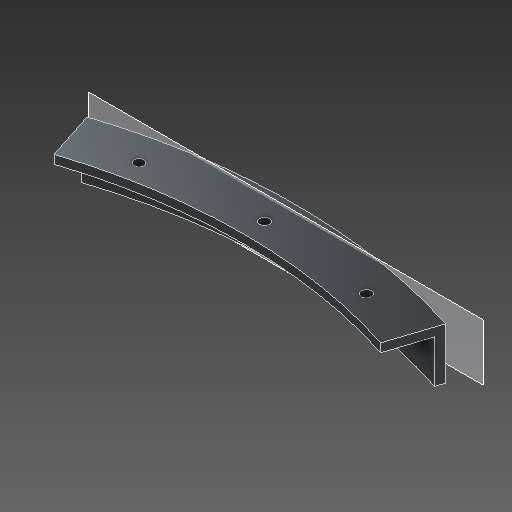
# Autodesk Inventor part: Casing_holder
Saved by Autodesk Inventor 2020 (Build 240168000, 168)
## iProperties
Created: 2022-08-25
Part Number: Casing_holder
Material: Iron, Gray Cast ASTM A48 Grade 60
Document SubType Name: Modeling
Designer: Umair
Density: 7.3953 g/cm^3
Appearance: Iron Gray
Author: Umair
Autodesk Inventor part; units mm, degrees
ref_plane "YZ Plane" through (0, 0, 0) normal (1, 0, 0) x (0, 1, 0)
ref_plane "XZ Plane" through (0, 0, 0) normal (0, 1, 0) x (-1, 0, 0)
sketch "Sketch1" plane through (0, 0, 0) normal (0, 1, 0) x (-1, 0, 0)
  circle A0 centre (0, 0) radius 200
  line L0 (0, 0) -> (0, -200)
  line L1 (0, 0) -> (-61.8034, -190.2113)
  line L2 (0, 0) -> (200, 0) construction
  line L3 (-61.8034, -190.2113) -> (0, 0)
  line L4 (0, 0) -> (61.8034, -190.2113)
  line L5 (0, 0) -> (200, 0) construction
  arc A1 (-61.8034, -190.2113) -> (61.8034, -190.2113) centre (0, 0) ccw
  line L6 (-61.8034, -190.2113) -> (-62.7304, -193.0645)
  line L7 (61.8034, -190.2113) -> (62.7304, -193.0645)
  line L8 (0, -200) -> (0, -203)
  arc A2 (-62.7304, -193.0645) -> (62.7304, -193.0645) centre (0, 0) ccw
  dimension "d0" = 400
  dimension "d1" = 108
  dimension "d2" = 72
  dimension "d4" = 3
  dimension "d5" = 3
  dimension "d6" = 3
  constraints: 18 end point, 9 point on circle, 3 centre point, 2 equal length, 2 horizontal, 2 vertical, 1 coincident, 1 collinear, 1 point on line
  measures "d0" diameter of A0
  measures "d1" angle of L1 L2
  measures "d2" angle of L4 L5
  measures "d4" distance of L1.end L6.end
  measures "d5" distance of L4.end L7.end
  measures "d6" distance of L0.end L8.end
extrude "Extrusion1" add sketch "Sketch1" along normal blind 3 and the other way blind 15 contours A0 L8 A2 L6 | L7 A2 L8 A0
sketch "Sketch3" plane through (0, 3, 0) normal (0, 1, 0) x (1, 0, 0)
  arc A0 (62.7304, 193.0645) -> (-62.7304, 193.0645) centre (0, 0) ccw projected
  line L0 (-62.7304, 193.0645) -> (-57.1681, 175.9455)
  line L1 (-62.7304, 193.0645) -> (-61.8034, 190.2113) projected
  line L2 (0, 203) -> (0, 185)
  line L3 (61.8034, 190.2113) -> (62.7304, 193.0645) projected
  line L4 (62.7304, 193.0645) -> (57.1681, 175.9455)
  arc A1 (57.1681, 175.9455) -> (-57.1681, 175.9455) centre (0, 0) ccw
  point P0 (0, 0)
  dimension "d12" = 18
  dimension "d13" = 18
  dimension "d14" = 18
  constraints: 6 end point, 4 point on circle, 2 collinear, 1 centre point, 1 vertical
  measures "d12" distance of L0.start L0.end
  measures "d13" distance of L2.start L2.end
  measures "d14" distance of L3.end L4.end
extrude "Extrusion2" add sketch "Sketch3" against normal blind 3
sketch "Sketch4" plane through (0, 3, 0) normal (0, 1, 0) x (1, 0, 0)
  arc A0 (62.7304, 193.0645) -> (-62.7304, 193.0645) centre (0, 0) ccw projected
  line L0 (0, 203) -> (0, 200)
  line L1 (0, 200) -> (0, 192.5)
  circle A1 centre (0, 192.5) radius 1.75
  line L2 (57.1681, 175.9455) -> (62.7304, 193.0645) projected
  line L3 (62.7304, 193.0645) -> (57.1681, 175.9455)
  line L4 (-62.7304, 193.0645) -> (-57.1681, 175.9455) projected
  line L5 (-62.7304, 193.0645) -> (-57.1681, 175.9455)
  line L6 (-57.1681, 175.9455) -> (-62.7304, 193.0645)
  line L7 (-62.7304, 193.0645) -> (-61.8034, 190.2113)
  line L8 (-61.8034, 190.2113) -> (-59.4858, 183.0784)
  line L9 (62.7304, 193.0645) -> (61.8034, 190.2113)
  line L10 (61.8034, 190.2113) -> (59.4858, 183.0784)
  arc A2 (59.4858, 183.0784) -> (-59.4858, 183.0784) centre (0, 0) ccw
  line L11 (0, 192.5) -> (39.7835, 188.3442)
  line L12 (39.7835, 188.3442) -> (0, 192.5)
  line L13 (0, 192.5) -> (-39.7835, 188.3442)
  circle A3 centre (39.7835, 188.3442) radius 1.75
  circle A4 centre (-39.7835, 188.3442) radius 1.75
  point P0 (0, 0)
  dimension "d17" = 3
  dimension "d18" = 7.5
  dimension "d19" = 3.5
  dimension "d28" = 3
  dimension "d29" = 7.5
  dimension "d30" = 3
  dimension "d31" = 7.5
  dimension "d32" = 40
  dimension "d33" = 40
  dimension "d34" = 3.5
  dimension "d35" = 3.5
  constraints: 24 end point, 6 point on circle, 5 point on line, 4 centre point, 3 coincident, 3 collinear, 1 vertical
  measures "d17" distance of L0.start L0.end
  measures "d18" distance of L0.end L1.end
  measures "d19" diameter of A1
  measures "d28" distance of L4.start L7.end
  measures "d29" distance of L7.end L8.end
  measures "d30" distance of L2.end L9.end
  measures "d31" distance of L9.end L10.end
  measures "d32" distance of L11.start L11.end
  measures "d33" distance of L11.start L13.end
  measures "d34" diameter of A3
  measures "d35" diameter of A4
extrude "Extrusion3" cut sketch "Sketch4" against normal blind 3 contours A1 A2 L1 | L1 A2 A1 | A3 L11 A2 | A2 A3 | L13 A1 A2 | A2 A1 L11 | L11 A1 L13 | L11 A3 A2 | A4 A2 | A2 L13 A4 | A4 L13 A2
ref_plane "Work Plane1" through (0, 0, -200) normal (0, 0, 1) x (1, 0, 0)
sketch "Sketch6" plane through (0, 0, -200) normal (0, 0, 1) x (1, 0, 0)
  line L0 (62.7304, 3) -> (-62.7304, 3) projected
  line L1 (0, 3) -> (0, -15)
  line L2 (-62.7304, -15) -> (62.7304, -15) projected
  line L3 (0, 3) -> (0, -15)
  line L4 (61.8034, -15) -> (-61.8034, -15) projected
  line L5 (0, 3) -> (0, 0)
  line L6 (0, 0) -> (0, -7.5)
  circle A0 centre (0, -7.5) radius 1.75
  line L7 (0, -7.5) -> (-40, -7.5)
  line L8 (-40, -7.5) -> (40, -7.5)
  circle A1 centre (-40, -7.5) radius 1.75
  circle A2 centre (40, -7.5) radius 1.75
  dimension "d23" = 3
  dimension "d24" = 7.5
  dimension "d25" = 3.5
  dimension "d36" = 40
  dimension "d37" = 80
  dimension "d38" = 3.5
  dimension "d39" = 3.5
  constraints: 12 end point, 3 centre point, 3 coincident, 2 midpoint, 2 point on line, 1 collinear, 1 horizontal, 1 perpendicular
  measures "d23" distance of L1.start L5.end
  measures "d24" distance of L5.end L6.end
  measures "d25" diameter of A0
  measures "d36" distance of L7.start L7.end
  measures "d37" distance of L7.end L8.end
  measures "d38" diameter of A1
  measures "d39" diameter of A2
extrude "Extrusion4" cut sketch "Sketch6" against normal mid plane 10
body "Solid1"
